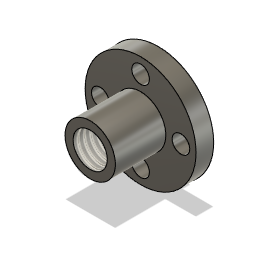
Brass+Nut (Autodesk Fusion 360 design; units mm, degrees)
Autodesk Fusion 360 part; units mm, degrees
note: some values were not read from the file. Set by a fixed rule: which face or edge a step refers to.
sketch "Sketch1" plane through (0, 0, 0) normal (0, 0, 1) x (1, 0, 0)
  circle A0 centre (0, 0) radius 11
  circle A1 centre (0, 0) radius 4
  circle A2 centre (0, 0) radius 5
  circle A3 centre (0, 0) radius 8 construction
  circle A4 centre (0, 8) radius 1.75
  circle A5 centre (-8, 0) radius 1.75
  circle A6 centre (0, -8) radius 1.75
  circle A7 centre (8, 0) radius 1.75
  dimension "d1" = 22
  dimension "d2" = 8
  dimension "d3" = 10
  dimension "d6" = 16
  dimension "d7" = 3.5
  dimension "d9" = 360
  constraint coincident A0.centre A1.centre
  constraint concentric A1 A2
  constraint coincident A3 A4.centre
  measures "d1" diameter of A0
  measures "d2" diameter of A1
  measures "d3" diameter of A2
  measures "d6" diameter of A3
  measures "d7" diameter of A4
extrude "Extrude1" add sketch "Sketch1" along normal blind 3.5 contours A0
extrude "Extrude2" add sketch "Sketch1" along normal blind 13.5 and the other way blind 1.5 contours A2
thread "Thread1" "ISO Metric profile 8.0 M8x1.25 6H" major diameter 8.17 minor diameter 6.7795 pitch 1.25 angle 60 resizes the face on face at (3.995, -0.1994, -1) on face at (3.995, -0.1994, 9)
